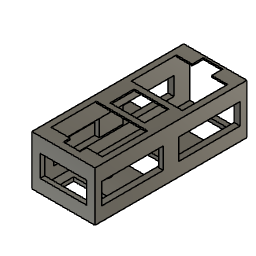
batteryCase (Autodesk Fusion 360 design; units mm, degrees)
Autodesk Fusion 360 part; units mm, degrees
sketch "Sketch1" plane through (0, 0, 0) normal (0, 0, 1) x (1, 0, 0)
  line L0 (21.65, 30) -> (-21.65, 30)
  line L1 (-21.65, 30) -> (-21.65, -30)
  line L2 (-21.65, -30) -> (21.65, -30)
  line L3 (21.65, -30) -> (21.65, 30) construction
  line L4 (21.65, 30) -> (-21.65, -30) construction
  line L5 (-21.65, 30) -> (21.65, -30) construction
  line L6 (0, 30) -> (0, -30) construction
  line L7 (21.65, 0) -> (-21.65, 0) construction
  circle A0 centre (-11.65, 20) radius 1.5
  circle A1 centre (11.65, 20) radius 1.5
  circle A2 centre (-11.65, -20) radius 1.5
  circle A3 centre (11.65, -20) radius 1.5
  line L8 (-6.5, 50.5) -> (35.5, 50.5)
  line L9 (35.5, 50.5) -> (35.5, -50.5)
  line L10 (35.5, -50.5) -> (-6.5, -50.5)
  line L11 (-6.5, -50.5) -> (-6.5, 50.5)
  line L12 (-6.5, 50.5) -> (35.5, -50.5) construction
  line L13 (35.5, 50.5) -> (-6.5, -50.5) construction
  line L14 (-6.5, 0) -> (35.5, 0) construction
  line L15 (31.5, 47.5) -> (-2.5, 47.5)
  line L16 (-2.5, 47.5) -> (-2.5, -47.5)
  line L17 (-2.5, -47.5) -> (31.5, -47.5)
  line L18 (31.5, -47.5) -> (31.5, 47.5)
  line L19 (31.5, 47.5) -> (-2.5, -47.5) construction
  line L20 (-2.5, 47.5) -> (31.5, -47.5) construction
  line L21 (-2.5, 47.5) -> (-2.5, 50.5)
  line L22 (31.5, 47.5) -> (31.5, 50.5)
  line L23 (14.5, 47.5) -> (14.5, -47.5) construction
  line L24 (-6.5, 16) -> (-10.5, 16)
  line L25 (-10.5, 16) -> (-10.5, 10)
  line L26 (-10.5, 10) -> (-6.5, 10)
  line L27 (-6.5, 10) -> (-6.5, 16)
  line L28 (-10.5, -10) -> (-6.5, -10)
  line L29 (-10.5, -16) -> (-10.5, -10)
  line L30 (-6.5, -16) -> (-10.5, -16)
  line L31 (11.65, 20) -> (-6.5, 20) construction
  line L32 (-6.5, 23.26) -> (-6.5, 16.3949)
  line L33 (-2.5, 17.3602) -> (-2.5, 22.9192)
  line L34 (-2.5, 22.9192) -> (-6.5, 16.3949) construction
  line L35 (-6.5, 23.26) -> (-2.5, 17.3602) construction
  line L36 (26, 32.2049) -> (3, 32.2049)
  line L37 (3, 32.2049) -> (3, 47.2049)
  line L38 (3, 47.2049) -> (26, 47.2049)
  line L39 (26, 47.2049) -> (26, 32.2049)
  line L40 (26, 32.2049) -> (3, 47.2049) construction
  line L41 (3, 32.2049) -> (26, 47.2049) construction
  line L42 (3, -47.2049) -> (26, -47.2049)
  line L43 (26, -32.2049) -> (3, -32.2049)
  line L44 (26, -47.2049) -> (26, -32.2049)
  line L45 (3, -32.2049) -> (3, -47.2049)
  line L46 (26, 7.5) -> (3, 7.5)
  line L47 (3, 7.5) -> (3, -7.5)
  line L48 (3, -7.5) -> (26, -7.5)
  line L49 (26, -7.5) -> (26, 7.5)
  line L50 (26, 7.5) -> (3, -7.5) construction
  line L51 (3, 7.5) -> (26, -7.5) construction
  point P0 (14.5, 0)
  point P1 (14.5, 0)
  point P2 (-4.2897, 20)
  point P3 (-4.2897, -20)
  point P4 (14.5, 0)
  point P5 (14.5, 39.7049)
  point P6 (14.5, 0)
  dimension "d1" = 43.3
  dimension "d2" = 60
  dimension "screwHoleThickness" = 3
  dimension "wSpacingScrew" = 11.65
  dimension "lSpacingScrew" = 20
  dimension "width" = 42
  dimension "lengthWall" = 101
  dimension "d8" = 34
  dimension "length" = 95
  dimension "d24" = 14.5
  dimension "screwwallcancel" = 4
  dimension "d26" = 6
  dimension "d27" = 10
  dimension "d43" = 23
  dimension "d44" = 15
  dimension "d45" = 23
  dimension "d46" = 15
  constraint horizontal L0
  constraint perpendicular L0 L1
  constraint parallel L0 L2
  constraint parallel L1 L3
  constraint coincident L4 origin
  constraint coincident L5 origin
  constraint midpoint L0 L6.start
  constraint midpoint L2 L6.end
  constraint midpoint L3 L7.start
  constraint midpoint L1 L7.end
  constraint symmetric L6 A0 A1
  constraint symmetric L7 A0 A2
  constraint symmetric L7 A1 A3
  constraint horizontal L8
  constraint perpendicular L8 L9
  constraint parallel L8 L10
  constraint parallel L9 L11
  constraint coincident L12 P6
  constraint coincident L13 P6
  constraint midpoint L11 L14.start
  constraint midpoint L9 L14.end
  constraint collinear L7 L14
  constraint horizontal L15
  constraint perpendicular L15 L16
  constraint parallel L15 L17
  constraint parallel L16 L18
  constraint coincident L19 P6
  constraint coincident L20 P6
  constraint coincident P6 P4
  constraint coincident L8 L21.end
  constraint perpendicular L8 L21
  constraint coincident L8 L22.end
  constraint perpendicular L8 L22
  constraint midpoint L15 L23.start
  constraint midpoint L17 L23.end
  constraint horizontal L24
  constraint vertical L25
  constraint horizontal L26
  constraint vertical L27
  constraint coincident L11 L24.start
  constraint symmetric L7 L24.start L30.start
  constraint symmetric L7 L24.end L29.start
  constraint symmetric L7 L25.end L28.start
  constraint symmetric L7 L26.end L28.end
  constraint coincident A1.centre L31.start
  constraint coincident L11 L31.end
  constraint perpendicular L11 L31
  constraint parallel L32 L33
  constraint coincident L16 L33.end
  constraint coincident L34 P2
  constraint coincident L35 P2
  constraint coincident L31 P2
  constraint collinear L11 L32
  constraint symmetric L14 P2 P3
  constraint horizontal L36
  constraint perpendicular L36 L37
  constraint parallel L36 L38
  constraint parallel L37 L39
  constraint coincident L40 P5
  constraint coincident L41 P5
  constraint coincident L23 P5
  constraint symmetric L7 L36.start L43.start
  constraint symmetric L7 L36.end L43.end
  constraint symmetric L7 L37.end L42.start
  constraint symmetric L7 L38.end L42.end
  constraint horizontal L46
  constraint perpendicular L46 L47
  constraint parallel L46 L48
  constraint parallel L47 L49
  constraint coincident L50 P6
  constraint coincident L51 P6
  measures "d1" distance of L1.end L2.end
  measures "d2" distance of L0.end L1.end
  measures "screwHoleThickness" diameter of A0
  measures "wSpacingScrew" distance of L6 A0.centre
  measures "lSpacingScrew" distance of L7 A0.centre
  measures "width" distance of L9.end L10.end
  measures "lengthWall" distance of L8.end L9.end
  measures "d8" distance of L16.end L17.end
  measures "length" distance of L15.end L16.end
  measures "d24" distance of L6 L23
  measures "screwwallcancel" distance of L24.start L24.end
  measures "d26" distance of L24.start L26.end
  measures "d27" distance of L7 L26
  measures "d43" distance of L37.end L38.end
  measures "d44" distance of L36.end L37.end
  measures "d45" distance of L47.end L48.end
  measures "d46" distance of L46.end L47.end
extrude "Extrude9" add sketch "Sketch1" along normal blind 2.5 contours L15 L16 L17 L18 L33 | L0 L1 L2 L11 L24 L25 L26 L28 L29 L30 L32 | L8 L15 L21 L22 makes body 1 at (-17.9333, -3.3333, 0) makes body 2 at (21.7167, 19.9016, 0)
extrude "Extrude10" add sketch "Sketch1" along normal blind 32 contours L0 L2 L11 L16 L27 L32 L33 | L0 L8 L11 L16 L21 | L2 L8 L9 L10 L11 L16 L17 L18 L22 bodies 1 2
sketch "Sketch2" plane through (35.5, 0, 0) normal (1, 0, 0) x (0, 1, 0)
  line L0 (-50.5, 0) -> (50.5, 0)
  line L1 (50.5, 0) -> (50.5, 32)
  line L2 (50.5, 32) -> (-50.5, 32)
  line L3 (-50.5, 32) -> (-50.5, 0)
  line L4 (0, 32) -> (0, 0) construction
  line L5 (50.5, 16) -> (-50.5, 16) construction
  line L6 (45.9932, 8.9649) -> (-45.9932, 8.9649)
  line L7 (-45.9932, 8.9649) -> (-45.9932, 23.0351)
  line L8 (-45.9932, 23.0351) -> (45.9932, 23.0351)
  line L9 (45.9932, 23.0351) -> (45.9932, 8.9649)
  line L10 (45.9932, 8.9649) -> (-45.9932, 23.0351) construction
  line L11 (-45.9932, 8.9649) -> (45.9932, 23.0351) construction
  line L12 (-5.1643, 23.0351) -> (-5.1643, 8.9649)
  line L13 (5.1722, 23.0351) -> (5.1722, 8.9649)
  point P0 (0, 16)
  constraint midpoint L2 L4.start
  constraint coincident L4.end origin
  constraint midpoint L1 L5.start
  constraint midpoint L3 L5.end
  constraint horizontal L6
  constraint perpendicular L6 L7
  constraint parallel L6 L8
  constraint parallel L7 L9
  constraint coincident L10 P0
  constraint coincident L11 P0
  constraint midpoint L4 P0
  constraint coincident L8 L12.start
  constraint coincident L6 L12.end
  constraint perpendicular L6 L12
  constraint coincident L8 L13.start
  constraint coincident L6 L13.end
  constraint perpendicular L6 L13
sketch "Sketch3" plane through (0, -50.5, 0) normal (0, -1, 0) x (1, 0, 0)
  line L0 (-6.5, 0) -> (35.5, 0)
  line L1 (35.5, 0) -> (35.5, 32)
  line L2 (35.5, 32) -> (-6.5, 32)
  line L3 (-6.5, 32) -> (-6.5, 0)
  line L4 (14.5, 32) -> (14.5, 0) construction
  line L5 (35.5, 16) -> (-6.5, 16) construction
  line L6 (29.9102, 8.8033) -> (-0.9102, 8.8033)
  line L7 (-0.9102, 8.8033) -> (-0.9102, 23.1967)
  line L8 (-0.9102, 23.1967) -> (29.9102, 23.1967)
  line L9 (29.9102, 23.1967) -> (29.9102, 8.8033)
  line L10 (29.9102, 8.8033) -> (-0.9102, 23.1967) construction
  line L11 (-0.9102, 8.8033) -> (29.9102, 23.1967) construction
  point P0 (14.5, 16)
  constraint midpoint L2 L4.start
  constraint midpoint L0 L4.end
  constraint midpoint L1 L5.start
  constraint midpoint L3 L5.end
  constraint horizontal L6
  constraint perpendicular L6 L7
  constraint parallel L6 L8
  constraint parallel L7 L9
  constraint coincident L10 P0
  constraint coincident L11 P0
  constraint midpoint L4 P0
extrude "Extrude11" cut sketch "Sketch3" against normal blind 3 contours L6 L7 L8 L9 bodies 1
extrude "Extrude12" cut sketch "Sketch2" against normal blind 4 contours L6 L8 L9 L13 | L6 L8 L12 L13 | L6 L7 L8 L12 bodies 1
sketch "Sketch4" plane through (-6.5, 0, 0) normal (-1, 0, 0) x (0, -1, 0)
  line L0 (-10, 0) -> (-10, 2.5)
  line L1 (-10, 2.5) -> (10, 2.5)
  line L2 (10, 2.5) -> (10, 0)
  line L3 (10, 0) -> (16, 0)
  line L4 (16, 0) -> (16, 2.5)
  line L5 (16, 2.5) -> (30, 2.5)
  line L6 (30, 2.5) -> (30, 0)
  line L7 (30, 0) -> (50.5, 0)
  line L8 (50.5, 0) -> (50.5, 32)
  line L9 (50.5, 32) -> (-50.5, 32)
  line L10 (-50.5, 32) -> (-50.5, 0)
  line L11 (-50.5, 0) -> (-30, 0)
  line L12 (-30, 0) -> (-30, 2.5)
  line L13 (-30, 2.5) -> (-16, 2.5)
  line L14 (-16, 2.5) -> (-16, 0)
  line L15 (-16, 0) -> (-10, 0)
  line L16 (0, 32) -> (0, 0) construction
  line L17 (50.5, 16) -> (-50.5, 16) construction
  line L18 (39.9916, 22.0397) -> (-39.9916, 22.0397)
  line L19 (-39.9916, 22.0397) -> (-39.9916, 9.9603)
  line L20 (-39.9916, 9.9603) -> (39.9916, 9.9603)
  line L21 (39.9916, 9.9603) -> (39.9916, 22.0397)
  line L22 (39.9916, 22.0397) -> (-39.9916, 9.9603) construction
  line L23 (-39.9916, 22.0397) -> (39.9916, 9.9603) construction
  line L24 (-7.0931, 22.0397) -> (8.6732, 22.0397)
  line L25 (8.6732, 22.0397) -> (8.6732, 9.9603)
  line L26 (8.6732, 9.9603) -> (-7.0931, 9.9603)
  line L27 (-7.0931, 9.9603) -> (-7.0931, 22.0397)
  point P0 (0, 16)
  constraint midpoint L9 L16.start
  constraint coincident L16.end origin
  constraint midpoint L8 L17.start
  constraint midpoint L10 L17.end
  constraint horizontal L18
  constraint perpendicular L18 L19
  constraint parallel L18 L20
  constraint parallel L19 L21
  constraint coincident L22 P0
  constraint coincident L23 P0
  constraint midpoint L17 P0
  constraint horizontal L24
  constraint vertical L25
  constraint horizontal L26
  constraint vertical L27
  constraint coincident L20 L25.end
  constraint coincident L18 L24.start
extrude "Extrude13" cut sketch "Sketch4" against normal blind 4 contours L18 L20 L21 L25 | L18 L20 L24 L25 L26 L27 | L18 L19 L20 L27 bodies 1
sketch "Sketch5" plane through (0, 0, 2.5) normal (0, 0, 1) x (-1, 0, 0)
  line L0 (-3, 47.2049) -> (-3, 32.2049)
  line L1 (-3, 32.2049) -> (-26, 32.2049)
  line L2 (-26, 32.2049) -> (-26, 47.2049)
  line L3 (-26, 47.2049) -> (-3, 47.2049)
  line L4 (-3, -47.2049) -> (-26, -47.2049)
  line L5 (-26, -47.2049) -> (-26, -32.2049)
  line L6 (-26, -32.2049) -> (-3, -32.2049)
  line L7 (-3, -32.2049) -> (-3, -47.2049)
  circle A0 centre (-11.65, -20) radius 1.5
  circle A1 centre (-11.65, 20) radius 1.5
  line L8 (-26, -7.5) -> (-26, 7.5)
  line L9 (-26, 7.5) -> (-3, 7.5)
  line L10 (-3, 7.5) -> (-3, -7.5)
  line L11 (-3, -7.5) -> (-26, -7.5)
  line L12 (2.5, 47.5) -> (-31.5, 47.5)
  line L13 (-31.5, 47.5) -> (-31.5, -50.5)
  line L14 (-31.5, -50.5) -> (2.5, -50.5)
  line L15 (2.5, -50.5) -> (2.5, 47.5)
  circle A2 centre (-11.65, -20) radius 4
  circle A3 centre (-11.65, 20) radius 4
  dimension "d57" = 8
  dimension "d58" = 8
  constraint concentric A0 A2
  constraint concentric A1 A3
  measures "d57" diameter of A2
  measures "d58" diameter of A3
extrude "Extrude14" cut sketch "Sketch5" against normal blind 0.5 contours A2 | A3 bodies 1
sketch "Sketch6" plane through (0, 0, 32) normal (0, 0, 1) x (-1, 0, 0)
  line L0 (2.5, 47.5) -> (2.5, -50.5)
  line L1 (2.5, -50.5) -> (6.5, -50.5)
  line L2 (6.5, -50.5) -> (6.5, 50.5)
  line L3 (6.5, 50.5) -> (-35.5, 50.5)
  line L4 (-35.5, 50.5) -> (-35.5, -50.5)
  line L5 (-35.5, -50.5) -> (-31.5, -50.5)
  line L6 (-31.5, -50.5) -> (-31.5, 47.5)
  line L7 (-31.5, 47.5) -> (2.5, 47.5)
  line L8 (6.5, -50.5) -> (-35.5, -50.5)
  line L9 (-35.5, -50.5) -> (-35.5, 50.5)
  line L10 (-35.5, 50.5) -> (6.5, 50.5)
  line L11 (6.5, 50.5) -> (6.5, -50.5)
  line L12 (2.5, -41.6336) -> (-31.5, -41.6336)
  line L13 (-31.5, -41.6336) -> (-31.5, -11.6336)
  line L14 (-31.5, -11.6336) -> (2.5, -11.6336)
  line L15 (2.5, -11.6336) -> (2.5, -41.6336)
  line L16 (2.5, 11.6067) -> (-31.5, 11.6067)
  line L17 (-31.5, 11.6067) -> (-31.5, 41.6067)
  line L18 (-31.5, 41.6067) -> (2.5, 41.6067)
  line L19 (2.5, 41.6067) -> (2.5, 11.6067)
  line L20 (-8, -49) -> (-21, -49)
  line L21 (-21, -49) -> (-21, -38)
  line L22 (-21, -38) -> (-8, -38)
  line L23 (-8, -38) -> (-8, -49)
  line L24 (-10, 37) -> (-21, 37)
  line L25 (-21, 37) -> (-21, 46)
  line L26 (-21, 46) -> (-10, 46)
  line L27 (-10, 46) -> (-10, 37)
  line L28 (2.5, -0.0134) -> (-31.5, -0.0134) construction
  line L29 (-3, -8) -> (-26, -8)
  line L30 (-26, -8) -> (-26, 8)
  line L31 (-26, 8) -> (-3, 8)
  line L32 (-3, 8) -> (-3, -8)
  dimension "d63" = 30
  dimension "d64" = 30
  constraint horizontal L8
  constraint vertical L9
  constraint horizontal L10
  constraint vertical L11
  constraint coincident L3.end L4.start
  constraint coincident L1.end L2.start
  constraint horizontal L12
  constraint vertical L13
  constraint horizontal L14
  constraint vertical L15
  constraint coincident L6 L13.end
  constraint coincident L0 L12.start
  constraint horizontal L16
  constraint vertical L17
  constraint horizontal L18
  constraint vertical L19
  constraint coincident L6 L17.end
  constraint coincident L0 L16.start
  constraint horizontal L20
  constraint vertical L21
  constraint horizontal L22
  constraint vertical L23
  constraint horizontal L24
  constraint vertical L25
  constraint horizontal L26
  constraint vertical L27
  constraint coincident L0 L28.start
  constraint coincident L6 L28.end
  constraint perpendicular L6 L28
  constraint symmetric L14 L16 L28
  constraint horizontal L29
  constraint vertical L30
  constraint horizontal L31
  constraint vertical L32
  measures "d63" distance of L16 L18
  measures "d64" distance of L12 L14
extrude "Extrude15" add sketch "Sketch6" along normal blind 1 contours L0 L1 L2 L3 L4 L5 L6 L7 L8 L9 L10 L11 L13 L15 L17 L19 | L0 L6 L7 L18 L25 L26 L27 | L0 L6 L14 L16 | L0 L6 L8 L12 L20 L21 L23 | L29 L30 L31 L32 bodies 1
extrude "Extrude16" cut sketch "Sketch6" along normal blind 2 contours L29 L30 L31 L32 bodies 1
extrude "Extrude17" add sketch "Sketch2" against normal blind 3 contours L6 L8 L12 L13 bodies 1
extrude "Extrude18" add sketch "Sketch4" against normal blind 3 contours L18 L20 L24 L25 L26 L27 bodies 1
extrude "Extrusion19" cut 2 faces at (8.5038, 20.2732, 2) (8.5038, -19.7268, 2) along direction (0, 0, -1) blind 0.5 on bodies 1 bodies 1
equation "d1 = 10 mm + 23.3 mm + 10 mm"
equation "d2 = 10 mm + 40 mm + 10 mm"
equation "width = 36 mm + 2 * wallThickness"
equation "lengthWall = length + 2 * wallThickness"
equation "wallThickness = 3 mm"
equation "zipHole = 6 mm"
equation "height = 32 mm"
